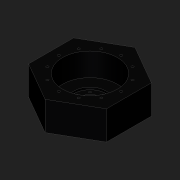
# Autodesk Inventor part: AC01
Saved by Autodesk Inventor 2017 (Build 210142000, 142)
## iProperties
Created: 2019-08-28
Part Number: AC01
Material: ABS Plastic
Document SubType Name: Modeling
Designer: Dell
Density: 1.06 g/cm^3
Appearance: Smooth - Black
Author: Dell
Autodesk Inventor part; units mm, degrees
ref_plane "YZ Plane" through (0, 0, 0) normal (1, 0, 0) x (0, 1, 0)
ref_plane "XZ Plane" through (0, 0, 0) normal (0, 1, 0) x (-1, 0, 0)
ref_plane "XY Plane" through (0, 0, 0) normal (0, 0, 1) x (1, 0, 0)
sketch "Sketch1" plane through (0, 0, 0) normal (0, 0, 1) x (1, 0, 0)
  circle A0 centre (0, 0) radius 17.5
  circle A1 centre (0, 0) radius 67.5
  circle A2 centre (22.5, 0) radius 2
  circle A3 centre (15.9099, 15.9099) radius 2
  circle A4 centre (0, 22.5) radius 2
  circle A5 centre (-15.9099, 15.9099) radius 2
  circle A6 centre (-22.5, 0) radius 2
  circle A7 centre (-15.9099, -15.9099) radius 2
  circle A8 centre (0, -22.5) radius 2
  circle A9 centre (15.9099, -15.9099) radius 2
  dimension "d0" = 35
  dimension "d1" = 135
  dimension "d2" = 4
  dimension "d3" = 22.5
  dimension "d6" = 360
  constraints: 10 centre point, 2 coincident, 1 horizontal alignment, 17 other
  measures "d0" diameter of A0
  measures "d1" diameter of A1
  measures "d2" diameter of A2
  measures "d3" distance of A2.centre point (0, 0)
extrude "Extrusion1" add sketch "Sketch1" along normal blind 10
sketch "Sketch5" plane through (0, 0, 10) normal (0, 0, 1) x (1, 0, 0)
  circle A0 centre (0, 0) radius 67.5 projected
  circle A1 centre (0, 0) radius 47.5
  dimension "d19" = 95
  constraints: 1 centre point
  measures "d19" diameter of A1
extrude "Extrusion4" add sketch "Sketch5" along normal blind 40
sketch "Sketch8" plane through (0, 0, 50) normal (0, 0, 1) x (1, 0, 0)
  circle A0 centre (-54, 0) radius 2
  circle A1 centre (-46.7654, -27) radius 2
  circle A2 centre (-27, -46.7654) radius 2
  circle A3 centre (0, -54) radius 2
  circle A4 centre (27, -46.7654) radius 2
  circle A5 centre (46.7654, -27) radius 2
  circle A6 centre (54, 0) radius 2
  circle A7 centre (46.7654, 27) radius 2
  circle A8 centre (27, 46.7654) radius 2
  circle A9 centre (0, 54) radius 2
  circle A10 centre (-27, 46.7654) radius 2
  circle A11 centre (-46.7654, 27) radius 2
  point P0 (0, 0)
  dimension "d20" = 4
  dimension "d21" = 54
  dimension "d24" = 360
  constraints: 12 centre point, 1 horizontal alignment, 25 other
  measures "d20" diameter of A0
  measures "d21" distance of point (0, 0) A0.centre
extrude "Extrusion5" cut sketch "Sketch8" against normal through all
sketch "Sketch9" plane through (0, 0, 10) normal (0, 0, 1) x (1, 0, 0)
  circle A0 centre (0, 0) radius 27.5
  dimension "d28" = 55
  constraints: 1 centre point, 1 coincident
  measures "d28" diameter of A0
extrude "Extrusion6" cut sketch "Sketch9" against normal blind 4
sketch "Sketch10" plane through (0, 0, 0) normal (0, 0, -1) x (-1, 0, 0)
  circle A0 centre (0, 0) radius 33
  circle A1 centre (0, 0) radius 47.5
  dimension "d31" = 66
  dimension "d32" = 95
  constraints: 2 centre point, 2 coincident
  measures "d31" diameter of A0
  measures "d32" diameter of A1
extrude "Extrusion7" cut sketch "Sketch10" against normal blind 5
sketch "Sketch11" plane through (0, 0, 50) normal (0, 0, 1) x (1, 0, 0)
  line L0 (0, 77.9423) -> (67.5, 38.9711)
  line L1 (67.5, 38.9711) -> (67.5, -38.9711)
  line L2 (67.5, -38.9711) -> (0, -77.9423)
  line L3 (0, -77.9423) -> (-67.5, -38.9711)
  line L4 (-67.5, -38.9711) -> (-67.5, 38.9711)
  line L5 (-67.5, 38.9711) -> (0, 77.9423)
  circle A0 centre (0, 0) radius 67.5 projected
  constraints: 12 end point, 1 coincident, 1 tangent, 1 vertical alignment, 13 other
extrude "Extrusion8" add sketch "Sketch11" against normal blind 50 contours L0 A0 L5 | L0 L1 A0 | A0 L4 L5 | L1 L2 A0 | A0 L3 L4 | L2 L3 A0
sketch "Sketch12" plane through (0, 0, 0) normal (0, 0, -1) x (-1, 0, 0)
  circle A0 centre (-54, 0) radius 2 projected
  circle A1 centre (-54, 0) radius 6.5
  circle A2 centre (-46.7654, -27) radius 6.5
  circle A3 centre (-27, -46.7654) radius 6.5
  circle A4 centre (0, -54) radius 6.5
  circle A5 centre (27, -46.7654) radius 6.5
  circle A6 centre (46.7654, -27) radius 6.5
  circle A7 centre (54, 0) radius 6.5
  circle A8 centre (46.7654, 27) radius 6.5
  circle A9 centre (27, 46.7654) radius 6.5
  circle A10 centre (0, 54) radius 6.5
  circle A11 centre (-27, 46.7654) radius 6.5
  circle A12 centre (-46.7654, 27) radius 6.5
  point P0 (0, 0)
  dimension "d37" = 13
  dimension "d40" = 360
  constraints: 12 centre point, 1 coincident, 25 other
  measures "d37" diameter of A1
extrude "Extrusion9" cut sketch "Sketch12" against normal blind 5 contours A0 | A1 | A2 | A3 | A4 | A5 | A6 | A7 | A8 | A9 | A10 | A11 | A12
sketch "Sketch14" plane through (0, 0, 0) normal (0, 0, -1) x (-1, 0, 0)
  circle A0 centre (-54, 0) radius 6.5 projected
  line L0 (-54, -6.5) -> (-47.0532, -6.5)
  line L1 (-47.0532, -6.5) -> (-47.0532, 6.5)
  line L2 (-47.0532, 6.5) -> (-54, 6.5)
  line L3 (-54, -6.5) -> (-54, 6.5)
  arc A1 (-47.5, 0) -> (-41.1362, -23.75) centre (0, 0) ccw projected
  line L4 (-43.5154, -32.6292) -> (-37.4992, -29.1557)
  line L5 (-37.4992, -29.1557) -> (-43.9992, -17.8974)
  line L6 (-43.9992, -17.8974) -> (-50.0154, -21.3708)
  line L7 (-43.5154, -32.6292) -> (-50.0154, -21.3708)
  line L8 (-21.3708, -50.0154) -> (-17.8974, -43.9992)
  line L9 (-17.8974, -43.9992) -> (-29.1557, -37.4992)
  line L10 (-29.1557, -37.4992) -> (-32.6292, -43.5154)
  line L11 (-21.3708, -50.0154) -> (-32.6292, -43.5154)
  line L12 (6.5, -54) -> (6.5, -47.0532)
  line L13 (6.5, -47.0532) -> (-6.5, -47.0532)
  line L14 (-6.5, -47.0532) -> (-6.5, -54)
  line L15 (6.5, -54) -> (-6.5, -54)
  line L16 (32.6292, -43.5154) -> (29.1557, -37.4992)
  line L17 (29.1557, -37.4992) -> (17.8974, -43.9992)
  line L18 (17.8974, -43.9992) -> (21.3708, -50.0154)
  line L19 (32.6292, -43.5154) -> (21.3708, -50.0154)
  line L20 (50.0154, -21.3708) -> (43.9992, -17.8974)
  line L21 (43.9992, -17.8974) -> (37.4992, -29.1557)
  line L22 (37.4992, -29.1557) -> (43.5154, -32.6292)
  line L23 (50.0154, -21.3708) -> (43.5154, -32.6292)
  line L24 (54, 6.5) -> (47.0532, 6.5)
  line L25 (47.0532, 6.5) -> (47.0532, -6.5)
  line L26 (47.0532, -6.5) -> (54, -6.5)
  line L27 (54, 6.5) -> (54, -6.5)
  line L28 (43.5154, 32.6292) -> (37.4992, 29.1557)
  line L29 (37.4992, 29.1557) -> (43.9992, 17.8974)
  line L30 (43.9992, 17.8974) -> (50.0154, 21.3708)
  line L31 (43.5154, 32.6292) -> (50.0154, 21.3708)
  line L32 (21.3708, 50.0154) -> (17.8974, 43.9992)
  line L33 (17.8974, 43.9992) -> (29.1557, 37.4992)
  line L34 (29.1557, 37.4992) -> (32.6292, 43.5154)
  line L35 (21.3708, 50.0154) -> (32.6292, 43.5154)
  line L36 (-6.5, 54) -> (-6.5, 47.0532)
  line L37 (-6.5, 47.0532) -> (6.5, 47.0532)
  line L38 (6.5, 47.0532) -> (6.5, 54)
  line L39 (-6.5, 54) -> (6.5, 54)
  line L40 (-32.6292, 43.5154) -> (-29.1557, 37.4992)
  line L41 (-29.1557, 37.4992) -> (-17.8974, 43.9992)
  line L42 (-17.8974, 43.9992) -> (-21.3708, 50.0154)
  line L43 (-32.6292, 43.5154) -> (-21.3708, 50.0154)
  line L44 (-50.0154, 21.3708) -> (-43.9992, 17.8974)
  line L45 (-43.9992, 17.8974) -> (-37.4992, 29.1557)
  line L46 (-37.4992, 29.1557) -> (-43.5154, 32.6292)
  line L47 (-50.0154, 21.3708) -> (-43.5154, 32.6292)
  dimension "d46" = 360
  constraints: 96 end point, 3 point on circle, 2 perpendicular, 2 tangent, 1 horizontal, 97 other
extrude "Extrusion10" cut sketch "Sketch14" against normal blind 5
body "Solid1"
